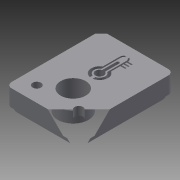
# Autodesk Inventor part: temperatura
Saved by Autodesk Inventor 2015 SP1 (Build 190203100, 203)
## iProperties
Created: 2015-07-05
Part Number: temperatura
Material: Genérico
Document SubType Name: Modeling
Designer: Javier
Density: 1 g/cm^3
Appearance: Valor por defecto
Author: Javier
Autodesk Inventor part; units mm, degrees
ref_plane "YZ Plane" through (0, 0, 0) normal (1, 0, 0) x (0, 1, 0)
ref_plane "XZ Plane" through (0, 0, 0) normal (0, 1, 0) x (-1, 0, 0)
ref_plane "XY Plane" through (0, 0, 0) normal (0, 0, 1) x (1, 0, 0)
sketch "Boceto1" plane through (0, 0, 0) normal (0, 0, 1) x (1, 0, 0)
  point P0 (0, 0)
sketch "Boceto2" plane through (0, 0, 0) normal (0, 0, 1) x (1, 0, 0)
  arc A0 (11.5, 13.5) -> (9.5, 15.5) centre (9.5, 13.5) ccw projected
  line L0 (9.5, 15.5) -> (-9.5, 15.5) projected
  arc A1 (-9.5, 15.5) -> (-11.5, 13.5) centre (-9.5, 13.5) ccw projected
  line L1 (-11.5, 13.5) -> (-11.5, -13.5) projected
  arc A2 (-11.5, -13.5) -> (-9.5, -15.5) centre (-9.5, -13.5) ccw projected
  line L2 (-9.5, -15.5) -> (9.5, -15.5) projected
  arc A3 (9.5, -15.5) -> (11.5, -13.5) centre (9.5, -13.5) ccw projected
  line L3 (11.5, -13.5) -> (11.5, 13.5) projected
  circle A4 centre (7.5, -11.5) radius 1.5 projected
  circle A5 centre (-7.5, -11.5) radius 1.5 projected
  line L4 (-4.5, 17.5) -> (-11.5, 17.5) projected
  arc A6 (-11.5, 17.5) -> (-13.5, 15.5) centre (-11.5, 15.5) ccw projected
  line L5 (-13.5, 15.5) -> (-13.5, -15.5) projected
  arc A7 (-13.5, -15.5) -> (-12.3012, -17.3325) centre (-11.5, -15.5) ccw projected
  arc A8 (-11.9943, -17.5) -> (-12.3012, -17.3325) centre (-13.1023, -19.165) ccw projected
  line L6 (11.9943, -17.5) -> (-11.9943, -17.5) projected
  arc A9 (12.3012, -17.3325) -> (11.9943, -17.5) centre (13.1023, -19.165) ccw projected
  arc A10 (12.3012, -17.3325) -> (13.5, -15.5) centre (11.5, -15.5) ccw projected
  line L7 (13.5, -15.5) -> (13.5, 15.5) projected
  arc A11 (13.5, 15.5) -> (11.5, 17.5) centre (11.5, 15.5) ccw projected
  line L8 (11.5, 17.5) -> (4.5, 17.5) projected
  line L9 (-4.5, 16.5) -> (-4.5, 17.5) projected
  line L10 (4.5, 17.5) -> (4.5, 16.5) projected
  line L11 (4.5, 16.5) -> (9.5, 16.5) projected
  arc A12 (12.5, 13.5) -> (9.5, 16.5) centre (9.5, 13.5) ccw projected
  line L12 (12.5, 13.5) -> (12.5, -13.5) projected
  arc A13 (9.5, -16.5) -> (12.5, -13.5) centre (9.5, -13.5) ccw projected
  line L13 (9.5, -16.5) -> (-9.5, -16.5) projected
  arc A14 (-12.5, -13.5) -> (-9.5, -16.5) centre (-9.5, -13.5) ccw projected
  line L14 (-12.5, -13.5) -> (-12.5, 13.5) projected
  arc A15 (-9.5, 16.5) -> (-12.5, 13.5) centre (-9.5, 13.5) ccw projected
  line L15 (-9.5, 16.5) -> (-4.5, 16.5) projected
  circle A16 centre (0, -6) radius 5.5 projected
  line L16 (-4.5, 15.5) -> (-4.5, 17.5)
  line L17 (4.5, 15.5) -> (4.5, 17.5)
  point P0 (0, 0)
  constraints: 4 end point, 2 point on line, 1 parallel, 1 vertical
extrude "Extrusión1" add sketch "Boceto2" along normal blind 3 contours A0 L0 L17 L11 A12 L12 A13 L13 A14 L14 A15 L15 L16 A1 L1 A2 L2 A3 L3 | L10 L8 A11 L7 A10 A9 L6 A8 A7 L5 A6 L4 L9 L15 A15 L14 A14 L13 A13 L12 A12 L11
sketch "Boceto3" plane through (0, 0, 3) normal (0, 0, 1) x (1, 0, 0)
  point P0 (0, 0)
lip "Labio1" kind lip height 1 width 1 edges at (11.5, 0, 0) (10.9142, -14.9142, 0) (0, -15.5, 0) (-10.9142, -14.9142, 0) (-11.5, 0, 0) (-10.9142, 14.9142, 0) (-7, 15.5, 0) (10.9142, 14.9142, 0) (7, 15.5, 0) guide face at (-12.8333, -4.5, 0)
sketch "Boceto4" plane through (0, 0, 3) normal (0, 0, 1) x (1, 0, 0)
  line L0 (-4.5, 17.5) -> (-11.5, 17.5) projected
  arc A0 (-11.5, 17.5) -> (-13.5, 15.5) centre (-11.5, 15.5) ccw projected
  line L1 (-13.5, 15.5) -> (-13.5, -15.5) projected
  arc A1 (-13.5, -15.5) -> (-12.3012, -17.3325) centre (-11.5, -15.5) ccw projected
  line L2 (-11.9943, -17.5) -> (11.9943, -17.5) projected
  arc A2 (12.3012, -17.3325) -> (13.5, -15.5) centre (11.5, -15.5) ccw projected
  line L3 (13.5, -15.5) -> (13.5, 15.5) projected
  arc A3 (13.5, 15.5) -> (11.5, 17.5) centre (11.5, 15.5) ccw projected
  line L4 (11.5, 17.5) -> (4.5, 17.5) projected
  line L5 (-4.5, 17.5) -> (4.5, 17.5)
  circle A4 centre (-7.5, -11.5) radius 1.5 projected
  circle A5 centre (7.5, -11.5) radius 1.5 projected
  line L6 (0, -15.5) -> (0, -6)
  circle A6 centre (0, -6) radius 4.5
  line L7 (12.3062, -17.3254) -> (11.9943, -17.5)
  arc A7 (12.3012, -17.3325) -> (11.9943, -17.5) centre (13.1023, -19.165) ccw projected
  line L8 (-12.3012, -17.3325) -> (-11.9943, -17.5)
  arc A8 (-11.9943, -17.5) -> (-12.3012, -17.3325) centre (-13.1023, -19.165) ccw projected
  dimension "d8" = 9.5
  dimension "d9" = 9
  constraints: 8 end point, 5 centre point, 1 coincident, 1 collinear, 1 vertical
  measures "d8" distance of L6.start L6.end
  measures "d9" diameter of A6
extrude "Extrusión2" add sketch "Boceto4" along normal blind 3 contours L5 L4 A3 L3 A2 A7 L2 A8 A1 L1 A0 L0
sketch "Boceto7" plane through (0, 0, 6) normal (0, 0, 1) x (1, 0, 0)
  arc A0 (-0.4971, 4.8605) -> (0.5107, 4.8605) centre (0.0068, 3.4352) ccw
  line L0 (0.5107, 9.9463) -> (0.5107, 4.8605)
  line L1 (-0.4971, 9.9463) -> (-0.4971, 4.8605)
  arc A1 (0.5107, 9.9463) -> (-0.4971, 9.9463) centre (0.0068, 9.9463) ccw
  line L2 (1.0186, 12.071) -> (1.0068, 5.1673)
  line L3 (-0.9932, 12.0744) -> (-0.9932, 5.1673)
  line L4 (-1.4932, 12.071) -> (-1.4932, 6.0333)
  line L5 (1.5186, 12.0651) -> (3.0194, 12.0651)
  line L6 (3.0186, 11.5651) -> (1.5186, 11.5676)
  line L7 (1.5186, 10.9496) -> (3.0194, 10.947)
  line L8 (3.0186, 10.447) -> (1.5186, 10.4496)
  line L9 (1.0158, 10.4547) -> (1.0148, 9.8367)
  line L10 (1.5186, 9.8316) -> (3.0194, 9.829)
  line L11 (3.0186, 9.329) -> (1.5186, 9.3316)
  arc A2 (3.0186, 11.5651) -> (3.0194, 12.0651) centre (3.019, 11.8151) ccw
  arc A3 (3.0186, 10.447) -> (3.0194, 10.947) centre (3.019, 10.697) ccw
  arc A4 (3.0186, 9.329) -> (3.0194, 9.829) centre (3.019, 9.579) ccw
  line L12 (1.5186, 9.3316) -> (1.5186, 6.0265)
  line L13 (1.5186, 11.5676) -> (1.5186, 10.9496)
  line L14 (1.5186, 10.4496) -> (1.5186, 9.8316)
  line L15 (0.5, 1.497) -> (0.5, 0.476)
  line L16 (-0.5, 1.5005) -> (-0.5, 0.4783)
  line L17 (-0.4843, 14.9619) -> (0.5157, 14.9619)
  line L18 (0.5157, 14.9619) -> (0.5157, 12.1919)
  line L19 (0.5157, 12.1919) -> (-0.4843, 12.1919)
  line L20 (-0.4843, 12.1919) -> (-0.4843, 14.9619)
  line L21 (-0.4843, 14.9619) -> (0.5157, 12.1919) construction
  line L22 (0.5157, 14.9619) -> (-0.4843, 12.1919) construction
  arc A5 (-0.9932, 5.1673) -> (-0.5, 1.5005) centre (0.0068, 3.4352) ccw
  arc A6 (0.5, 1.497) -> (1.0068, 5.1673) centre (0.0068, 3.4352) ccw
  arc A7 (-1.4932, 6.0333) -> (-0.5, 0.4783) centre (0.0068, 3.4352) ccw
  arc A8 (0.5, 0.476) -> (1.5186, 6.0265) centre (0.0068, 3.4352) ccw
  arc A9 (1.0186, 12.071) -> (0.5157, 12.9421) centre (0.0127, 12.071) ccw
  arc A10 (-0.4843, 12.9456) -> (-0.9932, 12.0744) centre (0.0127, 12.071) ccw
  arc A11 (1.5186, 12.0651) -> (0.5157, 13.4904) centre (0.0127, 12.071) ccw
  arc A12 (-0.4843, 13.4925) -> (-1.4932, 12.071) centre (0.0127, 12.071) ccw
  point P0 (0, 0)
  point P1 (-1.505, 3.4352)
  point P2 (0.0157, 13.5769)
  dimension "d31" = 0.618
  dimension "d35" = 1
  constraints: 46 end point, 28 point on circle, 13 centre point, 7 tangent, 6 point on line, 5 perpendicular, 3 coincident, 3 parallel, 2 horizontal, 2 midpoint
  measures "d31" distance of L9.start L9.end
  measures "d35" distance of L18.end L19.end
sketch "Boceto5" plane through (0, 0, 3) normal (0, 0, -1) x (-1, 0, 0)
  circle A0 centre (0, -6) radius 4.5 projected
  circle A1 centre (0, -6) radius 5.5
  point P0 (0, 0)
  dimension "d12" = 11
  constraints: 1 centre point, 1 coincident
  measures "d12" diameter of A1
extrude "Extrusión3" add sketch "Boceto5" along normal blind 4
sketch "Boceto6" plane through (0, 0, 6) normal (0, 0, 1) x (1, 0, 0)
  arc A0 (-12.3012, -17.3325) -> (-11.9943, -17.5) centre (-13.1023, -19.165) ccw projected
  arc A1 (11.9943, -17.5) -> (12.3012, -17.3325) centre (13.1023, -19.165) ccw projected
  circle A2 centre (-13.1023, -19.165) radius 2
  circle A3 centre (13.1023, -19.165) radius 2
  point P0 (0, 0)
  constraints: 2 centre point, 2 coincident, 2 concentric
extrude "Extrusión4" cut sketch "Boceto6" against normal blind 10
extrude "Extrusión5" cut sketch "Boceto7" against normal blind 10 contours L1 A1 L0 A0 | A9 L18 A11 L5 A2 L6 L13 L7 A3 L8 L14 L10 A4 L11 L12 A8 L15 A6 L2 | A10 L3 A5 L16 A7 L4 A12 L20
